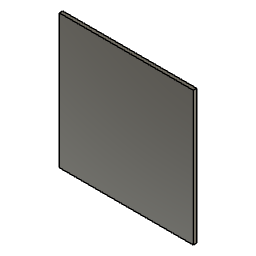
Woobly (Autodesk Fusion 360 design; units mm, degrees)
Autodesk Fusion 360 part; units mm, degrees
sketch "Sketch1" plane through (0, 0, 0) normal (0, 0, 1) x (1, 0, 0) in component "Mounting plate"
  line L0 (-67.3802, 0.9626) -> (52.6198, 0.9626)
  line L1 (52.6198, 0.9626) -> (52.6198, -2.0374)
  line L2 (52.6198, -2.0374) -> (-67.3802, -2.0374)
  line L3 (-67.3802, -2.0374) -> (-67.3802, 0.9626)
  dimension "d1" = 120
  dimension "d2" = 3
  constraint horizontal L0
  constraint vertical L1
  constraint horizontal L2
  constraint vertical L3
  measures "d1" distance of L1.end L2.end
  measures "d2" distance of L0.end L1.end
extrude "Extrude1" add sketch "Sketch1" along normal blind 120 in component "Mounting plate"
component "Mounting plate" placed x (1, 0, 0) y (0, 1, 0) z (0, 0, 1) at (0, 0, 0)
